Autodesk Inventor part; units mm, degrees
(part 2 of 2)
  line L511 (2.25, -360.25) -> (2.25, -339.75)
  line L512 (-2.25, -339.75) -> (-2.25, -360.25)
  arc A340 (-2.25, -360.25) -> (2.25, -360.25) centre (0, -360.25) ccw
  arc A341 (2.25, -339.75) -> (-2.25, -339.75) centre (0, -339.75) ccw
  line L513 (0, -325.25) -> (0, -304.75) construction
  line L514 (2.25, -325.25) -> (2.25, -304.75)
  line L515 (-2.25, -304.75) -> (-2.25, -325.25)
  arc A342 (-2.25, -325.25) -> (2.25, -325.25) centre (0, -325.25) ccw
  arc A343 (2.25, -304.75) -> (-2.25, -304.75) centre (0, -304.75) ccw
  line L516 (0, -290.25) -> (0, -269.75) construction
  line L517 (2.25, -290.25) -> (2.25, -269.75)
  line L518 (-2.25, -269.75) -> (-2.25, -290.25)
  arc A344 (-2.25, -290.25) -> (2.25, -290.25) centre (0, -290.25) ccw
  arc A345 (2.25, -269.75) -> (-2.25, -269.75) centre (0, -269.75) ccw
  line L519 (0, -255.25) -> (0, -234.75) construction
  line L520 (2.25, -255.25) -> (2.25, -234.75)
  line L521 (-2.25, -234.75) -> (-2.25, -255.25)
  arc A346 (-2.25, -255.25) -> (2.25, -255.25) centre (0, -255.25) ccw
  arc A347 (2.25, -234.75) -> (-2.25, -234.75) centre (0, -234.75) ccw
  line L522 (0, -220.25) -> (0, -199.75) construction
  line L523 (2.25, -220.25) -> (2.25, -199.75)
  line L524 (-2.25, -199.75) -> (-2.25, -220.25)
  arc A348 (-2.25, -220.25) -> (2.25, -220.25) centre (0, -220.25) ccw
  arc A349 (2.25, -199.75) -> (-2.25, -199.75) centre (0, -199.75) ccw
  line L525 (0, -185.25) -> (0, -164.75) construction
  line L526 (2.25, -185.25) -> (2.25, -164.75)
  line L527 (-2.25, -164.75) -> (-2.25, -185.25)
  arc A350 (-2.25, -185.25) -> (2.25, -185.25) centre (0, -185.25) ccw
  arc A351 (2.25, -164.75) -> (-2.25, -164.75) centre (0, -164.75) ccw
  line L528 (0, -150.25) -> (0, -129.75) construction
  line L529 (2.25, -150.25) -> (2.25, -129.75)
  line L530 (-2.25, -129.75) -> (-2.25, -150.25)
  arc A352 (-2.25, -150.25) -> (2.25, -150.25) centre (0, -150.25) ccw
  arc A353 (2.25, -129.75) -> (-2.25, -129.75) centre (0, -129.75) ccw
  line L531 (0, -115.25) -> (0, -94.75) construction
  line L532 (2.25, -115.25) -> (2.25, -94.75)
  line L533 (-2.25, -94.75) -> (-2.25, -115.25)
  arc A354 (-2.25, -115.25) -> (2.25, -115.25) centre (0, -115.25) ccw
  arc A355 (2.25, -94.75) -> (-2.25, -94.75) centre (0, -94.75) ccw
  line L534 (0, -80.25) -> (0, -59.75) construction
  line L535 (2.25, -80.25) -> (2.25, -59.75)
  line L536 (-2.25, -59.75) -> (-2.25, -80.25)
  arc A356 (-2.25, -80.25) -> (2.25, -80.25) centre (0, -80.25) ccw
  arc A357 (2.25, -59.75) -> (-2.25, -59.75) centre (0, -59.75) ccw
  line L537 (0, -45.25) -> (0, -24.75) construction
  line L538 (2.25, -45.25) -> (2.25, -24.75)
  line L539 (-2.25, -24.75) -> (-2.25, -45.25)
  arc A358 (-2.25, -45.25) -> (2.25, -45.25) centre (0, -45.25) ccw
  arc A359 (2.25, -24.75) -> (-2.25, -24.75) centre (0, -24.75) ccw
  line L540 (0, -10.25) -> (0, 10.25) construction
  line L541 (2.25, -10.25) -> (2.25, 10.25)
  line L542 (-2.25, 10.25) -> (-2.25, -10.25)
  arc A360 (-2.25, -10.25) -> (2.25, -10.25) centre (0, -10.25) ccw
  arc A361 (2.25, 10.25) -> (-2.25, 10.25) centre (0, 10.25) ccw
  line L543 (0, 24.75) -> (0, 45.25) construction
  line L544 (2.25, 24.75) -> (2.25, 45.25)
  line L545 (-2.25, 45.25) -> (-2.25, 24.75)
  arc A362 (-2.25, 24.75) -> (2.25, 24.75) centre (0, 24.75) ccw
  arc A363 (2.25, 45.25) -> (-2.25, 45.25) centre (0, 45.25) ccw
  line L546 (0, -465.25) -> (0, -444.75) construction
  line L547 (2.25, -465.25) -> (2.25, -444.75)
  line L548 (-2.25, -444.75) -> (-2.25, -465.25)
  arc A364 (-2.25, -465.25) -> (2.25, -465.25) centre (0, -465.25) ccw
  arc A365 (2.25, -444.75) -> (-2.25, -444.75) centre (0, -444.75) ccw
  line L549 (0, -430.25) -> (0, -409.75) construction
  line L550 (2.25, -430.25) -> (2.25, -409.75)
  line L551 (-2.25, -409.75) -> (-2.25, -430.25)
  arc A366 (-2.25, -430.25) -> (2.25, -430.25) centre (0, -430.25) ccw
  arc A367 (2.25, -409.75) -> (-2.25, -409.75) centre (0, -409.75) ccw
  line L552 (0, -395.25) -> (0, -374.75) construction
  line L553 (2.25, -395.25) -> (2.25, -374.75)
  line L554 (-2.25, -374.75) -> (-2.25, -395.25)
  arc A368 (-2.25, -395.25) -> (2.25, -395.25) centre (0, -395.25) ccw
  arc A369 (2.25, -374.75) -> (-2.25, -374.75) centre (0, -374.75) ccw
  line L555 (0, -360.25) -> (0, -339.75) construction
  line L556 (2.25, -360.25) -> (2.25, -339.75)
  line L557 (-2.25, -339.75) -> (-2.25, -360.25)
  arc A370 (-2.25, -360.25) -> (2.25, -360.25) centre (0, -360.25) ccw
  arc A371 (2.25, -339.75) -> (-2.25, -339.75) centre (0, -339.75) ccw
  line L558 (0, -325.25) -> (0, -304.75) construction
  line L559 (2.25, -325.25) -> (2.25, -304.75)
  line L560 (-2.25, -304.75) -> (-2.25, -325.25)
  arc A372 (-2.25, -325.25) -> (2.25, -325.25) centre (0, -325.25) ccw
  arc A373 (2.25, -304.75) -> (-2.25, -304.75) centre (0, -304.75) ccw
  line L561 (0, -290.25) -> (0, -269.75) construction
  line L562 (2.25, -290.25) -> (2.25, -269.75)
  line L563 (-2.25, -269.75) -> (-2.25, -290.25)
  arc A374 (-2.25, -290.25) -> (2.25, -290.25) centre (0, -290.25) ccw
  arc A375 (2.25, -269.75) -> (-2.25, -269.75) centre (0, -269.75) ccw
  line L564 (0, -255.25) -> (0, -234.75) construction
  line L565 (2.25, -255.25) -> (2.25, -234.75)
  line L566 (-2.25, -234.75) -> (-2.25, -255.25)
  arc A376 (-2.25, -255.25) -> (2.25, -255.25) centre (0, -255.25) ccw
  arc A377 (2.25, -234.75) -> (-2.25, -234.75) centre (0, -234.75) ccw
  line L567 (0, -220.25) -> (0, -199.75) construction
  line L568 (2.25, -220.25) -> (2.25, -199.75)
  line L569 (-2.25, -199.75) -> (-2.25, -220.25)
  arc A378 (-2.25, -220.25) -> (2.25, -220.25) centre (0, -220.25) ccw
  arc A379 (2.25, -199.75) -> (-2.25, -199.75) centre (0, -199.75) ccw
  line L570 (0, -185.25) -> (0, -164.75) construction
  line L571 (2.25, -185.25) -> (2.25, -164.75)
  line L572 (-2.25, -164.75) -> (-2.25, -185.25)
  arc A380 (-2.25, -185.25) -> (2.25, -185.25) centre (0, -185.25) ccw
  arc A381 (2.25, -164.75) -> (-2.25, -164.75) centre (0, -164.75) ccw
  line L573 (0, -150.25) -> (0, -129.75) construction
  line L574 (2.25, -150.25) -> (2.25, -129.75)
  line L575 (-2.25, -129.75) -> (-2.25, -150.25)
  arc A382 (-2.25, -150.25) -> (2.25, -150.25) centre (0, -150.25) ccw
  arc A383 (2.25, -129.75) -> (-2.25, -129.75) centre (0, -129.75) ccw
  line L576 (0, -115.25) -> (0, -94.75) construction
  line L577 (2.25, -115.25) -> (2.25, -94.75)
  line L578 (-2.25, -94.75) -> (-2.25, -115.25)
  arc A384 (-2.25, -115.25) -> (2.25, -115.25) centre (0, -115.25) ccw
  arc A385 (2.25, -94.75) -> (-2.25, -94.75) centre (0, -94.75) ccw
  line L579 (0, -80.25) -> (0, -59.75) construction
  line L580 (2.25, -80.25) -> (2.25, -59.75)
  line L581 (-2.25, -59.75) -> (-2.25, -80.25)
  arc A386 (-2.25, -80.25) -> (2.25, -80.25) centre (0, -80.25) ccw
  arc A387 (2.25, -59.75) -> (-2.25, -59.75) centre (0, -59.75) ccw
  line L582 (0, -45.25) -> (0, -24.75) construction
  line L583 (2.25, -45.25) -> (2.25, -24.75)
  line L584 (-2.25, -24.75) -> (-2.25, -45.25)
  arc A388 (-2.25, -45.25) -> (2.25, -45.25) centre (0, -45.25) ccw
  arc A389 (2.25, -24.75) -> (-2.25, -24.75) centre (0, -24.75) ccw
  line L585 (0, -10.25) -> (0, 10.25) construction
  line L586 (2.25, -10.25) -> (2.25, 10.25)
  line L587 (-2.25, 10.25) -> (-2.25, -10.25)
  arc A390 (-2.25, -10.25) -> (2.25, -10.25) centre (0, -10.25) ccw
  arc A391 (2.25, 10.25) -> (-2.25, 10.25) centre (0, 10.25) ccw
  line L588 (0, 479.75) -> (0, 500.25) construction
  line L589 (2.25, 479.75) -> (2.25, 500.25)
  line L590 (-2.25, 500.25) -> (-2.25, 479.75)
  arc A392 (-2.25, 479.75) -> (2.25, 479.75) centre (0, 479.75) ccw
  arc A393 (2.25, 500.25) -> (-2.25, 500.25) centre (0, 500.25) ccw
  line L591 (0, 444.75) -> (0, 465.25) construction
  line L592 (2.25, 444.75) -> (2.25, 465.25)
  line L593 (-2.25, 465.25) -> (-2.25, 444.75)
  arc A394 (-2.25, 444.75) -> (2.25, 444.75) centre (0, 444.75) ccw
  arc A395 (2.25, 465.25) -> (-2.25, 465.25) centre (0, 465.25) ccw
  line L594 (0, 409.75) -> (0, 430.25) construction
  line L595 (2.25, 409.75) -> (2.25, 430.25)
  line L596 (-2.25, 430.25) -> (-2.25, 409.75)
  arc A396 (-2.25, 409.75) -> (2.25, 409.75) centre (0, 409.75) ccw
  arc A397 (2.25, 430.25) -> (-2.25, 430.25) centre (0, 430.25) ccw
  line L597 (0, 374.75) -> (0, 395.25) construction
  line L598 (2.25, 374.75) -> (2.25, 395.25)
  line L599 (-2.25, 395.25) -> (-2.25, 374.75)
  arc A398 (-2.25, 374.75) -> (2.25, 374.75) centre (0, 374.75) ccw
  arc A399 (2.25, 395.25) -> (-2.25, 395.25) centre (0, 395.25) ccw
  line L600 (0, 339.75) -> (0, 360.25) construction
  line L601 (2.25, 339.75) -> (2.25, 360.25)
  line L602 (-2.25, 360.25) -> (-2.25, 339.75)
  arc A400 (-2.25, 339.75) -> (2.25, 339.75) centre (0, 339.75) ccw
  arc A401 (2.25, 360.25) -> (-2.25, 360.25) centre (0, 360.25) ccw
  line L603 (0, 304.75) -> (0, 325.25) construction
  line L604 (2.25, 304.75) -> (2.25, 325.25)
  line L605 (-2.25, 325.25) -> (-2.25, 304.75)
  arc A402 (-2.25, 304.75) -> (2.25, 304.75) centre (0, 304.75) ccw
  arc A403 (2.25, 325.25) -> (-2.25, 325.25) centre (0, 325.25) ccw
  line L606 (0, 269.75) -> (0, 290.25) construction
  line L607 (2.25, 269.75) -> (2.25, 290.25)
  line L608 (-2.25, 290.25) -> (-2.25, 269.75)
  arc A404 (-2.25, 269.75) -> (2.25, 269.75) centre (0, 269.75) ccw
  arc A405 (2.25, 290.25) -> (-2.25, 290.25) centre (0, 290.25) ccw
  line L609 (0, 234.75) -> (0, 255.25) construction
  line L610 (2.25, 234.75) -> (2.25, 255.25)
  line L611 (-2.25, 255.25) -> (-2.25, 234.75)
  arc A406 (-2.25, 234.75) -> (2.25, 234.75) centre (0, 234.75) ccw
  arc A407 (2.25, 255.25) -> (-2.25, 255.25) centre (0, 255.25) ccw
  line L612 (0, 199.75) -> (0, 220.25) construction
  line L613 (2.25, 199.75) -> (2.25, 220.25)
  line L614 (-2.25, 220.25) -> (-2.25, 199.75)
  arc A408 (-2.25, 199.75) -> (2.25, 199.75) centre (0, 199.75) ccw
  arc A409 (2.25, 220.25) -> (-2.25, 220.25) centre (0, 220.25) ccw
  line L615 (0, 164.75) -> (0, 185.25) construction
  line L616 (2.25, 164.75) -> (2.25, 185.25)
  line L617 (-2.25, 185.25) -> (-2.25, 164.75)
  arc A410 (-2.25, 164.75) -> (2.25, 164.75) centre (0, 164.75) ccw
  arc A411 (2.25, 185.25) -> (-2.25, 185.25) centre (0, 185.25) ccw
  line L618 (0, 129.75) -> (0, 150.25) construction
  line L619 (2.25, 129.75) -> (2.25, 150.25)
  line L620 (-2.25, 150.25) -> (-2.25, 129.75)
  arc A412 (-2.25, 129.75) -> (2.25, 129.75) centre (0, 129.75) ccw
  arc A413 (2.25, 150.25) -> (-2.25, 150.25) centre (0, 150.25) ccw
  line L621 (0, 94.75) -> (0, 115.25) construction
  line L622 (2.25, 94.75) -> (2.25, 115.25)
  line L623 (-2.25, 115.25) -> (-2.25, 94.75)
  arc A414 (-2.25, 94.75) -> (2.25, 94.75) centre (0, 94.75) ccw
  arc A415 (2.25, 115.25) -> (-2.25, 115.25) centre (0, 115.25) ccw
  line L624 (0, 59.75) -> (0, 80.25) construction
  line L625 (2.25, 59.75) -> (2.25, 80.25)
  line L626 (-2.25, 80.25) -> (-2.25, 59.75)
  arc A416 (-2.25, 59.75) -> (2.25, 59.75) centre (0, 59.75) ccw
  arc A417 (2.25, 80.25) -> (-2.25, 80.25) centre (0, 80.25) ccw
  line L627 (0, 24.75) -> (0, 45.25) construction
  line L628 (2.25, 24.75) -> (2.25, 45.25)
  line L629 (-2.25, 45.25) -> (-2.25, 24.75)
  arc A418 (-2.25, 24.75) -> (2.25, 24.75) centre (0, 24.75) ccw
  arc A419 (2.25, 45.25) -> (-2.25, 45.25) centre (0, 45.25) ccw
  line L630 (0, -500.25) -> (0, -479.75) construction
  line L631 (2.25, -500.25) -> (2.25, -479.75)
  line L632 (-2.25, -479.75) -> (-2.25, -500.25)
  arc A420 (-2.25, -500.25) -> (2.25, -500.25) centre (0, -500.25) ccw
  arc A421 (2.25, -479.75) -> (-2.25, -479.75) centre (0, -479.75) ccw
  line L633 (0, -465.25) -> (0, -444.75) construction
  line L634 (2.25, -465.25) -> (2.25, -444.75)
  line L635 (-2.25, -444.75) -> (-2.25, -465.25)
  arc A422 (-2.25, -465.25) -> (2.25, -465.25) centre (0, -465.25) ccw
  arc A423 (2.25, -444.75) -> (-2.25, -444.75) centre (0, -444.75) ccw
  line L636 (0, -430.25) -> (0, -409.75) construction
  line L637 (2.25, -430.25) -> (2.25, -409.75)
  line L638 (-2.25, -409.75) -> (-2.25, -430.25)
  arc A424 (-2.25, -430.25) -> (2.25, -430.25) centre (0, -430.25) ccw
  arc A425 (2.25, -409.75) -> (-2.25, -409.75) centre (0, -409.75) ccw
  line L639 (0, -395.25) -> (0, -374.75) construction
  line L640 (2.25, -395.25) -> (2.25, -374.75)
  line L641 (-2.25, -374.75) -> (-2.25, -395.25)
  arc A426 (-2.25, -395.25) -> (2.25, -395.25) centre (0, -395.25) ccw
  arc A427 (2.25, -374.75) -> (-2.25, -374.75) centre (0, -374.75) ccw
  line L642 (0, -360.25) -> (0, -339.75) construction
  line L643 (2.25, -360.25) -> (2.25, -339.75)
  line L644 (-2.25, -339.75) -> (-2.25, -360.25)
  arc A428 (-2.25, -360.25) -> (2.25, -360.25) centre (0, -360.25) ccw
  arc A429 (2.25, -339.75) -> (-2.25, -339.75) centre (0, -339.75) ccw
  line L645 (0, -325.25) -> (0, -304.75) construction
  line L646 (2.25, -325.25) -> (2.25, -304.75)
  line L647 (-2.25, -304.75) -> (-2.25, -325.25)
  arc A430 (-2.25, -325.25) -> (2.25, -325.25) centre (0, -325.25) ccw
  arc A431 (2.25, -304.75) -> (-2.25, -304.75) centre (0, -304.75) ccw
  line L648 (0, -290.25) -> (0, -269.75) construction
  line L649 (2.25, -290.25) -> (2.25, -269.75)
  line L650 (-2.25, -269.75) -> (-2.25, -290.25)
  arc A432 (-2.25, -290.25) -> (2.25, -290.25) centre (0, -290.25) ccw
  arc A433 (2.25, -269.75) -> (-2.25, -269.75) centre (0, -269.75) ccw
  line L651 (0, -255.25) -> (0, -234.75) construction
  line L652 (2.25, -255.25) -> (2.25, -234.75)
  line L653 (-2.25, -234.75) -> (-2.25, -255.25)
  arc A434 (-2.25, -255.25) -> (2.25, -255.25) centre (0, -255.25) ccw
  arc A435 (2.25, -234.75) -> (-2.25, -234.75) centre (0, -234.75) ccw
  line L654 (0, -220.25) -> (0, -199.75) construction
  line L655 (2.25, -220.25) -> (2.25, -199.75)
  line L656 (-2.25, -199.75) -> (-2.25, -220.25)
  arc A436 (-2.25, -220.25) -> (2.25, -220.25) centre (0, -220.25) ccw
  arc A437 (2.25, -199.75) -> (-2.25, -199.75) centre (0, -199.75) ccw
  line L657 (0, -185.25) -> (0, -164.75) construction
  line L658 (2.25, -185.25) -> (2.25, -164.75)
  line L659 (-2.25, -164.75) -> (-2.25, -185.25)
  arc A438 (-2.25, -185.25) -> (2.25, -185.25) centre (0, -185.25) ccw
  arc A439 (2.25, -164.75) -> (-2.25, -164.75) centre (0, -164.75) ccw
  line L660 (0, -150.25) -> (0, -129.75) construction
  line L661 (2.25, -150.25) -> (2.25, -129.75)
  line L662 (-2.25, -129.75) -> (-2.25, -150.25)
  arc A440 (-2.25, -150.25) -> (2.25, -150.25) centre (0, -150.25) ccw
  arc A441 (2.25, -129.75) -> (-2.25, -129.75) centre (0, -129.75) ccw
  line L663 (0, -115.25) -> (0, -94.75) construction
  line L664 (2.25, -115.25) -> (2.25, -94.75)
  line L665 (-2.25, -94.75) -> (-2.25, -115.25)
  arc A442 (-2.25, -115.25) -> (2.25, -115.25) centre (0, -115.25) ccw
  arc A443 (2.25, -94.75) -> (-2.25, -94.75) centre (0, -94.75) ccw
  line L666 (0, -80.25) -> (0, -59.75) construction
  line L667 (2.25, -80.25) -> (2.25, -59.75)
  line L668 (-2.25, -59.75) -> (-2.25, -80.25)
  arc A444 (-2.25, -80.25) -> (2.25, -80.25) centre (0, -80.25) ccw
  arc A445 (2.25, -59.75) -> (-2.25, -59.75) centre (0, -59.75) ccw
  line L669 (0, -45.25) -> (0, -24.75) construction
  line L670 (2.25, -45.25) -> (2.25, -24.75)
  line L671 (-2.25, -24.75) -> (-2.25, -45.25)
  arc A446 (-2.25, -45.25) -> (2.25, -45.25) centre (0, -45.25) ccw
  arc A447 (2.25, -24.75) -> (-2.25, -24.75) centre (0, -24.75) ccw
  line L672 (0, -10.25) -> (0, 10.25) construction
  line L673 (2.25, -10.25) -> (2.25, 10.25)
  line L674 (-2.25, 10.25) -> (-2.25, -10.25)
  arc A448 (-2.25, -10.25) -> (2.25, -10.25) centre (0, -10.25) ccw
  arc A449 (2.25, 10.25) -> (-2.25, 10.25) centre (0, 10.25) ccw
  point P0 (0, 0)
  point P1 (0, 35)
  point P2 (0, 70)
  point P3 (0, 105)
  point P4 (0, 140)
  point P5 (0, 175)
  point P6 (0, 210)
  point P7 (0, 245)
  point P8 (0, 280)
  point P9 (0, 315)
  point P10 (0, 350)
  point P11 (0, 385)
  point P12 (0, 420)
  point P13 (0, 455)
  point P14 (0, -35)
  point P15 (0, 0)
  point P16 (0, 35)
  point P17 (0, 70)
  point P18 (0, 105)
  point P19 (0, 140)
  point P20 (0, 175)
  point P21 (0, 210)
  point P22 (0, 245)
  point P23 (0, 280)
  point P24 (0, 315)
  point P25 (0, 350)
  point P26 (0, 385)
  point P27 (0, 420)
  point P28 (0, -70)
  point P29 (0, -35)
  point P30 (0, 0)
  point P31 (0, 35)
  point P32 (0, 70)
  point P33 (0, 105)
  point P34 (0, 140)
  point P35 (0, 175)
  point P36 (0, 210)
  point P37 (0, 245)
  point P38 (0, 280)
  point P39 (0, 315)
  point P40 (0, 350)
  point P41 (0, 385)
  point P42 (0, -105)
  point P43 (0, -70)
  point P44 (0, -35)
  point P45 (0, 0)
  point P46 (0, 35)
  point P47 (0, 70)
  point P48 (0, 105)
  point P49 (0, 140)
  point P50 (0, 175)
  point P51 (0, 210)
  point P52 (0, 245)
  point P53 (0, 280)
  point P54 (0, 315)
  point P55 (0, 350)
  point P56 (0, -140)
  point P57 (0, -105)
  point P58 (0, -70)
  point P59 (0, -35)
  point P60 (0, 0)
  point P61 (0, 35)
  point P62 (0, 70)
  point P63 (0, 105)
  point P64 (0, 140)
  point P65 (0, 175)
  point P66 (0, 210)
  point P67 (0, 245)
  point P68 (0, 280)
  point P69 (0, 315)
  point P70 (0, -175)
  point P71 (0, -140)
  point P72 (0, -105)
  point P73 (0, -70)
  point P74 (0, -35)
  point P75 (0, 0)
  point P76 (0, 35)
  point P77 (0, 70)
  point P78 (0, 105)
  point P79 (0, 140)
  point P80 (0, 175)
  point P81 (0, 210)
  point P82 (0, 245)
  point P83 (0, 280)
  point P84 (0, -210)
  point P85 (0, -175)
  point P86 (0, -140)
  point P87 (0, -105)
  point P88 (0, -70)
  point P89 (0, -35)
  point P90 (0, 0)
  point P91 (0, 35)
  point P92 (0, 70)
  point P93 (0, 105)
  point P94 (0, 140)
  point P95 (0, 175)
  point P96 (0, 210)
  point P97 (0, 245)
  point P98 (0, -245)
  point P99 (0, -210)
  point P100 (0, -175)
  point P101 (0, -140)
  point P102 (0, -105)
  point P103 (0, -70)
  point P104 (0, -35)
  point P105 (0, 0)
  point P106 (0, 35)
  point P107 (0, 70)
  point P108 (0, 105)
  point P109 (0, 140)
  point P110 (0, 175)
  point P111 (0, 210)
  point P112 (0, -280)
  point P113 (0, -245)
  point P114 (0, -210)
  point P115 (0, -175)
  point P116 (0, -140)
  point P117 (0, -105)
  point P118 (0, -70)
  point P119 (0, -35)
  point P120 (0, 0)
  point P121 (0, 35)
  point P122 (0, 70)
  point P123 (0, 105)
  point P124 (0, 140)
  point P125 (0, 175)
  point P126 (0, -315)
  point P127 (0, -280)
  point P128 (0, -245)
  point P129 (0, -210)
  point P130 (0, -175)
  point P131 (0, -140)
  point P132 (0, -105)
  point P133 (0, -70)
  point P134 (0, -35)
  point P135 (0, 0)
  point P136 (0, 35)
  point P137 (0, 70)
  point P138 (0, 105)
  point P139 (0, 140)
  point P140 (0, -350)
  point P141 (0, -315)
  point P142 (0, -280)
  point P143 (0, -245)
  point P144 (0, -210)
  point P145 (0, -175)
  point P146 (0, -140)
  point P147 (0, -105)
  point P148 (0, -70)
  point P149 (0, -35)
  point P150 (0, 0)
  point P151 (0, 35)
  point P152 (0, 70)
  point P153 (0, 105)
  point P154 (0, -385)
  point P155 (0, -350)
  point P156 (0, -315)
  point P157 (0, -280)
  point P158 (0, -245)
  point P159 (0, -210)
  point P160 (0, -175)
  point P161 (0, -140)
  point P162 (0, -105)
  point P163 (0, -70)
  point P164 (0, -35)
  point P165 (0, 0)
  point P166 (0, 35)
  point P167 (0, 70)
  point P168 (0, -420)
  point P169 (0, -385)
  point P170 (0, -350)
  point P171 (0, -315)
  point P172 (0, -280)
  point P173 (0, -245)
  point P174 (0, -210)
  point P175 (0, -175)
  point P176 (0, -140)
  point P177 (0, -105)
  point P178 (0, -70)
  point P179 (0, -35)
  point P180 (0, 0)
  point P181 (0, 35)
  point P182 (0, -455)
  point P183 (0, -420)
  point P184 (0, -385)
  point P185 (0, -350)
  point P186 (0, -315)
  point P187 (0, -280)
  point P188 (0, -245)
  point P189 (0, -210)
  point P190 (0, -175)
  point P191 (0, -140)
  point P192 (0, -105)
  point P193 (0, -70)
  point P194 (0, -35)
  point P195 (0, 0)
  point P196 (0, 490)
  point P197 (0, 455)
  point P198 (0, 420)
  point P199 (0, 385)
  dimension "d23" = 10.25
  dimension "d24" = 4.5
  dimension "d27" = 35
  dimension "d30" = 35
  constraints: 1800 end point, 900 point on circle, 450 centre point, 4 tangent, 3 vertical, 2 collinear, 1 midpoint, 1 parallel, 2686 other
  measures "d23" distance of point (0, 0) L0.end
  measures "d24" diameter of A1
  measures "d27" distance of point (0, 0) point (0, 35)
  measures "d30" distance of point (0, 0) point (0, -35)
extrude "Cut1" cut sketch "Sketch4" against normal blind 1.5
equation "\"d33\" = Thickness"
equation "\"d2\" = Thickness"
equation "\"d3\" = BendReliefWidth"
equation "\"d4\" = BendReliefDepth"
equation "\"d5\" = MinimumRemnant"
equation "\"d6\" = TransitionRadius"
equation "\"d9\" = BendRadius"
equation "\"d10\" = CornerReliefSize"
equation "\"d11\" = GapSize"
equation "\"d12\" = JacobiRadiusSize"
equation "\"d13\" = BendReliefWidth"
equation "\"d14\" = BendReliefDepth"
equation "\"d15\" = MinimumRemnant"
equation "\"d16\" = TransitionRadius"
equation "\"d19\" = BendRadius"
equation "\"d20\" = CornerReliefSize"
equation "\"d21\" = GapSize"
equation "\"d22\" = JacobiRadiusSize"
equation "\"BendRadius\" = Thickness"
equation "\"BendReliefWidth\" = Thickness"
equation "\"BendReliefDepth\" = 0.5 * Thickness"
equation "\"CornerReliefSize\" = 4 * Thickness"
equation "\"MinimumRemnant\" = 2 * Thickness"
equation "\"TransitionRadius\" = BendRadius"
equation "\"JacobiRadiusSize\" = BendRadius"
equation "\"GapSize\" = Thickness"
equation "\"Thickness\" = 1.5"
body "Solid1"
